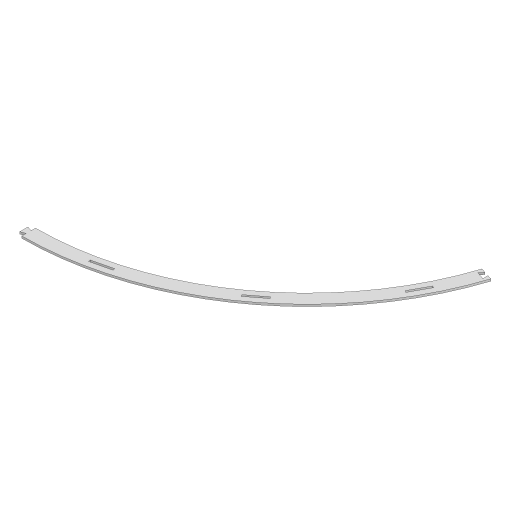
# Autodesk Inventor part: R80_CM_CIRCULO
Saved by Autodesk Inventor 2024.2 (Build 282272000, 272)
## iProperties
Created: 2024-10-01
Part Number: R80_CM_CIRCULO
Material: Generic
Document SubType Name: Modeling
Designer: jrcer
Density: 1 g/cm^3
Appearance: Default
Author: jrcer
Autodesk Inventor part; units mm, degrees
ref_plane "YZ Plane" through (0, 0, 0) normal (1, 0, 0) x (0, 1, 0)
ref_plane "XZ Plane" through (0, 0, 0) normal (0, 1, 0) x (-1, 0, 0)
ref_plane "XY Plane" through (0, 0, 0) normal (0, 0, 1) x (1, 0, 0)
sketch "Sketch1" plane through (0, 0, 0) normal (0, 1, 0) x (-1, 0, 0)
  circle A0 centre (0, 0) radius 400
  circle A1 centre (0, 0) radius 420
  line L0 (420, 0) -> (400, 0)
  line L1 (-420, 0) -> (-400, 0)
  line L2 (0, 0) -> (-380.4226, 123.6068) construction
  line L3 (0, 400) -> (0, 0) construction
  line L4 (0, 420) -> (0, 400)
  line L5 (-380.4226, 123.6068) -> (-399.4437, 129.7871)
  line L6 (-382.0637, 131.5003) -> (-393.4764, 135.2085)
  line L7 (-393.4764, 135.2085) -> (-393.2164, 127.7638)
  line L8 (-382.0637, 131.5003) -> (-386.6499, 125.6302)
  line L9 (-389.9332, 126.697) -> (-387.7701, 133.3544) construction
  line L10 (-368.6664, 183.0267) -> (-354.3558, 209.3935)
  line L11 (-354.3558, 209.3935) -> (-351.5434, 207.867)
  line L12 (-351.5434, 207.867) -> (-365.8539, 181.5003)
  line L13 (-365.8539, 181.5003) -> (-368.6664, 183.0267)
  line L14 (-368.6664, 183.0267) -> (-351.5434, 207.867) construction
  line L15 (-354.3558, 209.3935) -> (-365.8539, 181.5003) construction
  circle A2 centre (0, 0) radius 410 construction
  line L16 (-243.1284, -322.7284) -> (-238.9628, -328.9041)
  line L17 (-250.1818, -332.4366) -> (-243.0211, -334.4899)
  line L18 (-243.1284, -322.7284) -> (-250.1818, -332.4366)
  line L19 (231.8021, -330.9574) -> (238.9628, -328.9041)
  line L20 (238.8555, -340.6656) -> (243.0211, -334.4899)
  line L21 (231.8021, -330.9574) -> (238.8555, -340.6656)
  line L22 (386.39, 118.1855) -> (386.6499, 125.6302)
  line L23 (397.8026, 121.8937) -> (393.2164, 127.7638)
  line L24 (386.39, 118.1855) -> (397.8026, 121.8937)
  line L25 (7, 404) -> (0, 406.5478)
  line L26 (7, 416) -> (0, 413.4522)
  line L27 (7, 404) -> (7, 416)
  line L28 (-411.2372, 17.2531) -> (-408.8882, 47.161)
  line L29 (-408.047, 17.0025) -> (-411.2372, 17.2531)
  line L30 (-405.698, 46.9104) -> (-408.047, 17.0025)
  line L31 (-408.8882, 47.161) -> (-405.698, 46.9104)
  line L32 (-382.7013, -151.5037) -> (-392.72, -123.2261)
  line L33 (-379.685, -150.4351) -> (-382.7013, -151.5037)
  line L34 (-389.7037, -122.1574) -> (-379.685, -150.4351)
  line L35 (-392.72, -123.2261) -> (-389.7037, -122.1574)
  line L36 (-287.9929, -294.0642) -> (-308.647, -272.3062)
  line L37 (-285.6721, -291.8611) -> (-287.9929, -294.0642)
  line L38 (-306.3262, -270.1031) -> (-285.6721, -291.8611)
  line L39 (-308.647, -272.3062) -> (-306.3262, -270.1031)
  line L40 (-143.488, -385.7783) -> (-171.2062, -374.3022)
  line L41 (-142.2638, -382.8217) -> (-143.488, -385.7783)
  line L42 (-169.982, -371.3456) -> (-142.2638, -382.8217)
  line L43 (-171.2062, -374.3022) -> (-169.982, -371.3456)
  line L44 (25.8274, -410.7878) -> (-4.1622, -411.5779)
  line L45 (25.7431, -407.5889) -> (25.8274, -410.7878)
  line L46 (-4.2465, -408.379) -> (25.7431, -407.5889)
  line L47 (-4.1622, -411.5779) -> (-4.2465, -408.379)
  line L48 (190.677, -364.7684) -> (163.6015, -377.688)
  line L49 (189.2989, -361.8803) -> (190.677, -364.7684)
  line L50 (162.2234, -374.8) -> (189.2989, -361.8803)
  line L51 (163.6015, -377.688) -> (162.2234, -374.8)
  line L52 (322.5567, -255.6772) -> (303.0769, -278.4925)
  line L53 (320.1231, -253.5994) -> (322.5567, -255.6772)
  line L54 (300.6433, -276.4146) -> (320.1231, -253.5994)
  line L55 (303.0769, -278.4925) -> (300.6433, -276.4146)
  line L56 (398.6635, -102.3771) -> (390.1476, -131.143)
  line L57 (395.5952, -101.4687) -> (398.6635, -102.3771)
  line L58 (387.0793, -130.2347) -> (395.5952, -101.4687)
  line L59 (390.1476, -131.143) -> (387.0793, -130.2347)
  line L60 (405.8378, 68.6249) -> (409.7583, 38.8822)
  line L61 (402.6652, 68.2067) -> (405.8378, 68.6249)
  line L62 (406.5857, 38.464) -> (402.6652, 68.2067)
  line L63 (409.7583, 38.8822) -> (406.5857, 38.464)
  line L64 (342.839, 227.7611) -> (358.518, 202.1844)
  line L65 (340.1108, 226.0887) -> (342.839, 227.7611)
  line L66 (355.7898, 200.5119) -> (340.1108, 226.0887)
  line L67 (358.518, 202.1844) -> (355.7898, 200.5119)
  line L68 (220.5602, 347.5153) -> (245.2867, 330.527)
  line L69 (218.7481, 344.8778) -> (220.5602, 347.5153)
  line L70 (243.4746, 327.8895) -> (218.7481, 344.8778)
  line L71 (245.2867, 330.527) -> (243.4746, 327.8895)
  line L72 (60.1446, 407.1809) -> (89.6431, 401.7186)
  line L73 (59.5619, 404.0344) -> (60.1446, 407.1809)
  line L74 (89.0604, 398.572) -> (59.5619, 404.0344)
  line L75 (89.6431, 401.7186) -> (89.0604, 398.572)
  line L76 (-110.6706, 396.4413) -> (-81.5006, 403.4493)
  line L77 (-109.9231, 393.3298) -> (-110.6706, 396.4413)
  line L78 (-80.7531, 400.3378) -> (-109.9231, 393.3298)
  line L79 (-81.5006, 403.4493) -> (-80.7531, 400.3378)
  line L80 (-262.3498, 317.1534) -> (-238.5521, 335.42)
  line L81 (-260.4014, 314.6149) -> (-262.3498, 317.1534)
  line L82 (-236.6037, 332.8816) -> (-260.4014, 314.6149)
  line L83 (-238.5521, 335.42) -> (-236.6037, 332.8816)
  point P0 (410, 0)
  point P1 (-410, 0)
  point P2 (-360.1049, 195.4469)
  point P3 (-78.3853, 402.4372)
  point P4 (-367.2602, 182.2635)
  point P5 (-352.9496, 208.6303)
  point P6 (-246.6551, -327.5825)
  point P7 (235.3288, -335.8115)
  point P8 (392.0963, 120.0396)
  point P9 (7, 410)
  point P10 (-409.6421, 17.1278)
  point P11 (-407.2931, 47.0357)
  point P12 (-381.1932, -150.9694)
  point P13 (-391.2119, -122.6917)
  point P14 (-286.8325, -292.9626)
  point P15 (-307.4866, -271.2047)
  point P16 (-142.8759, -384.3)
  point P17 (-170.5941, -372.8239)
  point P18 (25.7853, -409.1884)
  point P19 (-4.2043, -409.9784)
  point P20 (189.9879, -363.3244)
  point P21 (162.9124, -376.244)
  point P22 (321.3399, -254.6383)
  point P23 (301.8601, -277.4536)
  point P24 (397.1293, -101.9229)
  point P25 (388.6135, -130.6889)
  point P26 (404.2515, 68.4158)
  point P27 (408.172, 38.6731)
  point P28 (341.4749, 226.9249)
  point P29 (357.1539, 201.3482)
  point P30 (219.6542, 346.1965)
  point P31 (244.3807, 329.2083)
  point P32 (59.8533, 405.6077)
  point P33 (89.3518, 400.1453)
  point P34 (-110.2968, 394.8856)
  point P35 (-81.1269, 401.8936)
  point P36 (-261.3756, 315.8841)
  point P37 (-237.5779, 334.1508)
  dimension "d0" = 800
  dimension "d1" = 840
  dimension "d4" = 72
  dimension "d5" = 7
  dimension "d6" = 70
  dimension "d8" = 12
  dimension "d13" = 3.2
  dimension "d14" = 30
  dimension "d15" = 50
  dimension "d20" = 820
  dimension "d23" = 360
  dimension "d27" = 360
  constraints: 168 end point, 11 point on circle, 8 midpoint, 3 centre point, 3 coincident, 3 parallel, 2 horizontal, 2 horizontal alignment, 2 perpendicular, 2 point on line, 2 vertical, 1 collinear, 1 equal length, 192 other
  measures "d0" diameter of A0
  measures "d1" diameter of A1
  measures "d4" angle of L2 L3
  measures "d5" distance between parallel lines of L6 L5
  measures "d6" angle of L7 L6
  measures "d8" distance of L6.start L6.end
  measures "d13" distance of L10.end L11.end
  measures "d14" distance of L11.end L12.end
  measures "d15" vertical distance of L12.end L6.start
  measures "d20" diameter of A2
extrude "Extrusion1" add sketch "Sketch1" along normal blind 3 contours A0 L5 L8 L6 L7 A1 L4 | L4 L26 L27 L25
body "Solid1"
